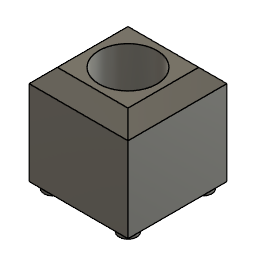
Proyecto control (Autodesk Fusion 360 design; units mm, degrees)
Autodesk Fusion 360 part; units mm, degrees
box "CajaPrimitiva1" add length 70 width 70 height 70 placed x (0, 0, -1) y (-1, 0, 0) z (0, 1, 0) at (10, 0, 55) makes body 1
move_body "Desplazar2" bodies 1 to x (1, 0, 0) y (0, 1, 0) z (0, 0, 1) at (10, -2, 0)
hole "Agujero1" at (-15, 68, 20) direction (0, -1, 0) diameter 34 depth 40 tip angle 180 counterbore diameter 41 counterbore depth 30 bodies 1
move_body "Desplazar3" bodies 1 to x (1, 0, 0) y (0, 1, 0) z (0, 0, 1) at (0, 10, 0)
cylinder "CilindroPrimitivo1" add diameter 12.659 height 5 placed x (1, 0, 0) y (0, 0, 1) z (0, -1, 0) at (-39.0753, 8, 44.4735) separate body makes body 2
move_body "Desplazar4" bodies 2 1 to x (1, 0, 0) y (0, 1, 0) z (0, 0, 1) at (-0.2337, 0, -5.9487)
move_body "Desplazar5" bodies 2 to x (1, 0, 0) y (0, 1, 0) z (0, 0, 1) at (-1.3787, 0.4245, 1.1292)
move_body "Desplazar18" bodies 2 to x (1, 0, 0) y (0, 1, 0) z (0, 0, 1) at (-1.0673, 0.2059, 0.9495)
pattern_linear "Patrón R1" count 2 spacing 53 along (0, 0, -1) count 2 spacing 53 along (1, 0, 0) of bodies 2 makes body 3 at (-35.457, 5.2971, -13.0267) makes body 4 at (17.543, 5.2971, 39.9733) makes body 5 at (17.543, 5.2971, -13.0267)
combine "Combinar1" operation add target body 1 tool bodies 5
combine "Combinar2" operation add target body 1 tool bodies 4 3 2
box "CajaPrimitiva2" add length 41 width 41 height 30 placed x (0, 0, -1) y (-1, 0, 0) z (0, 1, 0) at (25, 0, 25) separate body makes body 6
move_body "Desplazar19" bodies 6 to x (1, 0, 0) y (0, 1, 0) z (0, 0, 1) at (-19.3084, -35, 9.4542)
move_body "Desplazar20" bodies 1 to x (1, 0, 0) y (0, 1, 0) z (0, 0, 1) at (15.2337, -8, -14.0513)
move_body "Desplazar21" bodies 6 to x (1, 0, 0) y (0, 1, 0) z (0, 0, 1) at (14.8084, 35, -13.9542)
combine "Combinar3" operation cut target body 1 tool bodies 6
chamfer "Chaflán1" distance 10 angle 45 4 edges at (35, 70, 0) (0, 70, -35) (0, 70, 35) (-35, 70, 0) tangent chain off on bodies 1
